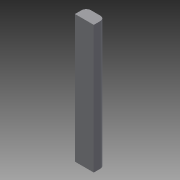
# Autodesk Inventor part: BumperSide
Saved by Autodesk Inventor 2013 (Build 170138000, 138)
## iProperties
Created: 2014-01-09
Part Number: BumperSide
Material: Generic
Document SubType Name: Modeling
Designer: 215152
Density: 1 g/cm^3
Author: 215152
Autodesk Inventor part; units mm, degrees
ref_plane "YZ Plane" through (0, 0, 0) normal (1, 0, 0) x (0, 1, 0)
ref_plane "XZ Plane" through (0, 0, 0) normal (0, 1, 0) x (-1, 0, 0)
ref_plane "XY Plane" through (0, 0, 0) normal (0, 0, 1) x (1, 0, 0)
sketch "Sketch1" plane through (0, 0, 0) normal (0, 0, 1) x (1, 0, 0)
  line L0 (0, 0) -> (127, 0)
  line L1 (127, 0) -> (127, 76.2)
  line L2 (127, 76.2) -> (0, 76.2)
  line L3 (0, 76.2) -> (0, 0)
  line L4 (127, 76.2) -> (0, 76.2)
  line L5 (0, 76.2) -> (0, -889)
  line L6 (0, -889) -> (127, -889)
  line L7 (127, -889) -> (127, 76.2)
  dimension "d0" = 127
  dimension "d1" = 76.2
  dimension "d2" = 127
  dimension "d3" = 965.2
  constraints: 16 end point, 4 parallel, 2 horizontal, 2 perpendicular
  measures "d0" distance of L2.end L1.end
  measures "d1" distance of L1.end L0.end
  measures "d2" distance of L6.end L5.end
  measures "d3" distance of L5.end L4.end
extrude "Extrusion1" add sketch "Sketch1" along normal blind 76.2
fillet "Fillet1" radius 31.75 2 edges at (127, -406.4, 0) (0, -406.4, 0)
sketch "Sketch2" plane through (0, 76.2, 76.2) normal (0, 1, 0) x (1, 0, 0)
  arc A0 (31.75, 76.2) -> (0, 44.45) centre (31.75, 44.45) ccw projected
  line L0 (0, 44.45) -> (0, 0) projected
  line L1 (127, 0) -> (0, 0) projected
  line L2 (127, 44.45) -> (127, 0) projected
  arc A1 (127, 44.45) -> (95.25, 76.2) centre (95.25, 44.45) ccw projected
  line L3 (95.25, 76.2) -> (31.75, 76.2) projected
  point P0 (0, 76.2)
extrude "Extrusion2" cut sketch "Sketch2" against normal blind 101.6
body "Solid1"
